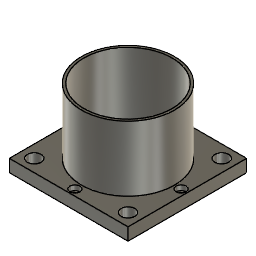
OpenATC-Base-bottom-cover (Autodesk Fusion 360 design; units mm, degrees)
Autodesk Fusion 360 part; units mm, degrees
sketch "Sketch1" plane through (0, 0, 0) normal (0, 0, 1) x (1, 0, 0)
  line L0 (-47.5, 47.5) -> (47.5, 47.5)
  line L1 (47.5, 47.5) -> (47.5, -47.5)
  line L2 (47.5, -47.5) -> (-47.5, -47.5)
  line L3 (-47.5, -47.5) -> (-47.5, 47.5)
  line L4 (-47.5, 47.5) -> (47.5, -47.5) construction
  line L5 (-47.5, -47.5) -> (47.5, 47.5) construction
  circle A0 centre (0, 0) radius 35.2
  dimension "d1" = 95
  dimension "d2" = 95
  dimension "d3" = 70.4
  constraint horizontal L0
  constraint vertical L1
  constraint horizontal L2
  constraint vertical L3
  constraint coincident A0.centre L4
  constraint coincident A0.centre L5
  constraint coincident A0.centre origin
  measures "d1" distance of L1.end L2.end
  measures "d2" distance of L0.start L2.end
  measures "d3" diameter of A0
extrude "Extrude1" add sketch "Sketch1" along normal blind 10
sketch "Sketch2" plane through (0, 0, 10) normal (0, 0, 1) x (-1, 0, 0)
  circle A0 centre (0, 0) radius 35.2
  line L0 (47.5, 47.5) -> (-47.5, 47.5)
  line L1 (-47.5, 47.5) -> (-47.5, -47.5)
  line L2 (-47.5, -47.5) -> (47.5, -47.5)
  line L3 (47.5, -47.5) -> (47.5, 47.5)
  line L4 (42.5, 0) -> (-42.5, 0) construction
  line L5 (0, -42.5) -> (0, 42.5) construction
  point P0 (0, -42.5)
  point P1 (42.5, 0)
  point P2 (0, 42.5)
  point P3 (-42.5, 0)
  dimension "d7" = 5
  dimension "d8" = 5
  dimension "d9" = 5
  dimension "d10" = 5
  constraint coincident P1 L4.start
  constraint coincident P3 L4.end
  constraint coincident P0 L5.start
  constraint coincident P2 L5.end
  constraint perpendicular L0 L5
  constraint horizontal L4
  constraint coincident A0.centre L4
  constraint coincident A0.centre L5
  measures "d7" distance of L0 P2
  measures "d8" distance of L3 P1
  measures "d9" distance of L1 P3
  measures "d10" distance of L2 P0
hole "Hole1" at (-42.5, 0, 10) at (0, 42.5, 10) at (42.5, 0, 10) at (0, -42.5, 10) direction (0, 0, -1) diameter 4.5 depth 15 tip angle 118 counterbore diameter 8 counterbore depth 4
sketch "Sketch3" plane through (0, 0, 10) normal (0, 0, 1) x (-1, 0, 0)
  circle A0 centre (-42.5, 0) radius 4
  circle A1 centre (42.5, 0) radius 4
  circle A2 centre (0, -42.5) radius 4
  circle A3 centre (0, 42.5) radius 4
  circle A4 centre (0, 0) radius 35.2
  line L0 (47.5, 47.5) -> (-47.5, 47.5)
  line L1 (-47.5, 47.5) -> (-47.5, -47.5)
  line L2 (-47.5, -47.5) -> (47.5, -47.5)
  line L3 (47.5, -47.5) -> (47.5, 47.5)
  circle A5 centre (0, 0) radius 35.2
  circle A6 centre (0, 0) radius 37.2
  dimension "d16" = 2
  constraint concentric A4 A5
  constraint concentric A5 A6
  constraint tangent A4 A5
  measures "d16" distance of A5 A6
extrude "Extrude2" add sketch "Sketch3" along normal blind 52 contours A6
sketch "Sketch4" plane through (0, 0, 10) normal (0, 0, 1) x (-1, 0, 0)
  circle A0 centre (0, 0) radius 37.2
  circle A1 centre (-42.5, 0) radius 4
  circle A2 centre (42.5, 0) radius 4
  circle A3 centre (0, -42.5) radius 4
  circle A4 centre (0, 42.5) radius 4
  line L0 (47.5, 47.5) -> (-47.5, 47.5)
  line L1 (-47.5, 47.5) -> (-47.5, -47.5)
  line L2 (-47.5, -47.5) -> (47.5, -47.5)
  line L3 (47.5, -47.5) -> (47.5, 47.5)
  line L4 (37.5, -37.5) -> (-37.5, -37.5) construction
  line L5 (-37.5, -37.5) -> (-37.5, 37.5) construction
  line L6 (-37.5, 37.5) -> (37.5, 37.5) construction
  line L7 (37.5, 37.5) -> (37.5, -37.5) construction
  point P0 (37.5, -37.5)
  point P1 (-37.5, -37.5)
  point P2 (-37.5, 37.5)
  point P3 (37.5, 37.5)
  dimension "d19" = 10
  dimension "d20" = 10
  dimension "d21" = 10
  dimension "d22" = 10
  constraint horizontal L4
  constraint vertical L5
  constraint horizontal L6
  constraint vertical L7
  constraint coincident P0 L4.start
  constraint coincident P1 L4.end
  constraint coincident P2 L5.end
  constraint coincident P3 L6.end
  measures "d19" distance of L0 L6
  measures "d20" distance of L3 L7
  measures "d21" distance of L2 L4
  measures "d22" distance of L1 L5
hole "Hole2" at (-37.5, -37.5, 10) at (-37.5, 37.5, 10) at (37.5, 37.5, 10) at (37.5, -37.5, 10) direction (0, 0, -1) diameter 11 end through all
equation "d2 = d1"
equation "d8 = d7"
equation "d9 = d7"
equation "d10 = d7"
equation "d20 = d19"
equation "d21 = d19"
equation "d22 = d19"
